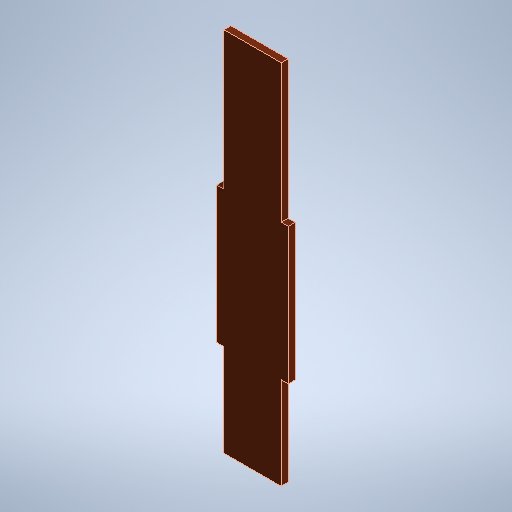
# Autodesk Inventor part: Motor Fixation .2
Saved by Autodesk Inventor 2025.4 (Build 294407000, 407)
## iProperties
Created: 2026-04-06
Part Number: Motor Fixation .2
Material: Generic
Document SubType Name: Sheet Metal
Designer: lenovo
Density: 1 g/cm^3
Sheet Metal Rule: Default_mm
Appearance: Default(1)
Author: lenovo
Autodesk Inventor part; units mm, degrees
ref_plane "YZ Plane" through (0, 0, 0) normal (1, 0, 0) x (0, 1, 0)
ref_plane "XZ Plane" through (0, 0, 0) normal (0, 1, 0) x (-1, 0, 0)
ref_plane "XY Plane" through (0, 0, 0) normal (0, 0, 1) x (1, 0, 0)
sketch "Sketch1" plane through (0, 0, 0) normal (0, 0, 1) x (1, 0, 0)
  line L0 (-12.5, -70) -> (12.5, -70)
  line L1 (12.5, -70) -> (12.5, 70)
  line L2 (12.5, 70) -> (-12.5, 70)
  line L3 (-12.5, 70) -> (-12.5, -70)
  line L4 (-12.5, -70) -> (12.5, 70) construction
  line L5 (12.5, -70) -> (-12.5, 70) construction
  line L6 (0, 70) -> (0, -70)
  line L7 (12.5, 29.75) -> (15.6, 29.75)
  line L8 (15.6, 29.75) -> (15.6, -29.75)
  line L9 (15.6, -29.75) -> (12.5, -29.75)
  line L10 (12.5, -29.75) -> (12.5, 29.75)
  line L11 (-12.5, 29.75) -> (-15.6, 29.75)
  line L12 (-15.6, 29.75) -> (-15.6, -29.75)
  line L13 (-15.6, -29.75) -> (-12.5, -29.75)
  line L14 (-12.5, -29.75) -> (-12.5, 29.75)
  line L15 (-12.5, 70) -> (12.5, 70)
  line L16 (12.5, 70) -> (12.5, 90)
  line L17 (12.5, 90) -> (-12.5, 90)
  line L18 (-12.5, 90) -> (-12.5, 70)
  point P0 (0, 0)
  point P1 (15.6, 0)
  point P2 (0, 0)
  point P3 (-15.6, 0)
  point P4 (-12.5, 29.75)
  point P5 (-12.5, -29.75)
  point P6 (12.5, -29.75)
  dimension "d0" = 140
  dimension "d1" = 59.5
  dimension "d2" = 3.1
  dimension "d3" = 25
  dimension "d5" = 20
  measures "d0" distance of L0.end L1.end
  measures "d1" distance of L7.end L8.end
  measures "d2" distance of L8.end L9.end
  measures "d3" distance of L1.end L2.end
  measures "d5" distance of L15.end L16.end
extrude "Plate1" add sketch "Sketch1" along normal mid plane 3
equation "\"d4\" = Thickness"
equation "\"BendRadius\" = Thickness"
equation "\"BendReliefWidth\" = Thickness"
equation "\"BendReliefDepth\" = 0.5 * Thickness"
equation "\"CornerReliefSize\" = 4 * Thickness"
equation "\"MinimumRemnant\" = 2 * Thickness"
equation "\"TransitionRadius\" = BendRadius"
equation "\"JacobiRadiusSize\" = BendRadius"
equation "\"GapSize\" = Thickness"
equation "\"Thickness\" = 3"
body "Solid1"
